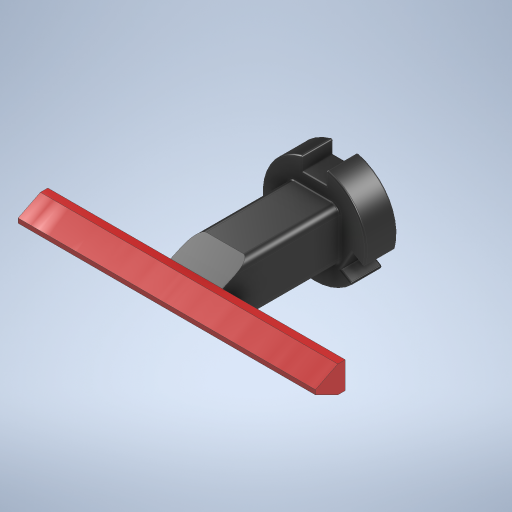
# Autodesk Inventor part: Squeegee
Saved by Autodesk Inventor 2023 (Build 270158000, 158)
## iProperties
Created: 2022-09-20
Part Number: Squeegee
Material: Generic
Document SubType Name: Modeling
Designer: benni
Density: 1 g/cm^3
Appearance: Default
Author: benni
Autodesk Inventor part; units mm, degrees
ref_plane "YZ Plane" through (0, 0, 0) normal (1, 0, 0) x (0, 1, 0)
ref_plane "XZ Plane" through (0, 0, 0) normal (0, 1, 0) x (-1, 0, 0)
ref_plane "XY Plane" through (0, 0, 0) normal (0, 0, 1) x (1, 0, 0)
sketch "Sketch1" plane through (0, 0, 0) normal (0, 0, 1) x (1, 0, 0)
  circle A0 centre (0, 0) radius 25 construction
  line L0 (0, 0) -> (0, 25) construction
  line L1 (0, 0) -> (21.6506, -12.5) construction
  line L2 (0, 0) -> (-21.6506, -12.5) construction
  line L3 (0, 25) -> (8, 25)
  line L4 (0, 25) -> (-8, 25)
  line L5 (0, 25) -> (8, 25) construction
  line L6 (21.6506, -12.5) -> (25.6506, -5.5718)
  line L7 (21.6506, -12.5) -> (29.6506, -12.5) construction
  line L8 (21.6506, -12.5) -> (17.6506, -19.4282)
  line L9 (21.6506, -12.5) -> (29.6506, -12.5) construction
  line L10 (-21.6506, -12.5) -> (-25.6506, -5.5718)
  line L11 (-21.6506, -12.5) -> (-13.6506, -12.5) construction
  line L12 (-21.6506, -12.5) -> (-17.6506, -19.4282)
  line L13 (-21.6506, -12.5) -> (-13.6506, -12.5) construction
  line L14 (8, 25) -> (8, 34.0735)
  line L15 (-8, 25) -> (-8, 34.0735)
  line L16 (25.6506, -5.5718) -> (33.5085, -10.1085)
  line L17 (17.6506, -19.4282) -> (25.5085, -23.9649)
  line L18 (-17.6506, -19.4282) -> (-25.5085, -23.9649)
  line L19 (-25.6506, -5.5718) -> (-33.5085, -10.1085)
  arc A1 (33.5085, -10.1085) -> (8, 34.0735) centre (0, 0) ccw
  arc A2 (-8, 34.0735) -> (-33.5085, -10.1085) centre (0, 0) ccw
  arc A3 (-25.5085, -23.9649) -> (25.5085, -23.9649) centre (0, 0) ccw
  dimension "d0" = 50
  dimension "d1" = 120
  dimension "d2" = 120
  dimension "d3" = 8
  dimension "d4" = 8
  dimension "d5" = 180
  dimension "d6" = 8
  dimension "d7" = 60
  dimension "d8" = 8
  dimension "d9" = 120
  dimension "d10" = 8
  dimension "d11" = 120
  dimension "d12" = 8
  dimension "d13" = 60
  dimension "d15" = 35
  dimension "d16" = 35
  dimension "d17" = 35
  constraints: 40 end point, 9 point on circle, 6 horizontal, 5 equal length, 4 centre point, 4 tangent, 3 parallel, 2 coincident, 2 perpendicular, 2 vertical, 1 collinear
  measures "d0" diameter of A0
  measures "d1" angle of L1 L0
  measures "d2" angle of L2 L1
  measures "d3" distance of L0.end L3.end
  measures "d4" distance of L0.end L4.end
  measures "d5" angle of L4 L5
  measures "d6" distance of L1.end L6.end
  measures "d7" angle of L7 L6
  measures "d8" distance of L1.end L8.end
  measures "d9" angle of L8 L9
  measures "d10" distance of L2.end L10.end
  measures "d11" angle of L11 L10
  measures "d12" distance of L2.end L12.end
  measures "d13" angle of L12 L13
  measures "d15" radius of A1
  measures "d16" radius of A2
  measures "d17" radius of A3
extrude "Extrusion1" add sketch "Sketch1" along normal blind 21
sketch "Sketch2" plane through (0, 0, 21) normal (0, 0, 1) x (1, 0, 0)
  line L0 (-17.5, -17.5) -> (17.5, -17.5)
  line L1 (17.5, -17.5) -> (17.5, 17.5)
  line L2 (17.5, 17.5) -> (-17.5, 17.5)
  line L3 (-17.5, 17.5) -> (-17.5, -17.5)
  line L4 (-17.5, -17.5) -> (17.5, 17.5) construction
  line L5 (17.5, -17.5) -> (-17.5, 17.5) construction
  point P0 (0, 0)
  dimension "d20" = 35
  dimension "d21" = 35
  constraints: 12 end point, 2 midpoint, 2 parallel, 1 horizontal, 1 perpendicular
  measures "d20" distance of L2.end L1.end
  measures "d21" distance of L1.end L0.end
extrude "Extrusion2" add sketch "Sketch2" along normal blind 79
fillet "Fillet1" radius 5 4 edges at (17.5, 17.5, 60.5) (17.5, -17.5, 60.5) (-17.5, 17.5, 60.5) (-17.5, -17.5, 60.5)
fillet "Fillet2" radius 1 37 edges at (30.3109, 17.5, 0) (-30.3109, 17.5, 0) (0, -35, 0) (21.6506, -12.5, 0) (29.5796, -7.8402, 0) (21.5796, -21.6966, 0) (8, 29.5367, 0) (0, 25, 0) (-8, 29.5367, 0) (-29.5796, -7.8402, 0) (-21.6506, -12.5, 0) (-21.5796, -21.6966, 0) (16.0355, 16.0355, 21) (17.5, 0, 21) (16.0355, -16.0355, 21) (0, -17.5, 21) (-16.0355, -16.0355, 21) (-17.5, 0, 21) (-16.0355, 16.0355, 21) (0, 17.5, 21) (0, 25, 21) (8, 29.5367, 21) (30.3109, 17.5, 21) (8, 34.0735, 10.5) (-8, 34.0735, 10.5) (-30.3109, 17.5, 21) (21.6506, -12.5, 21) (29.5796, -7.8402, 21) (33.5085, -10.1085, 10.5) (21.5796, -21.6966, 21) (25.5085, -23.9649, 10.5) (0, -35, 21) (-21.5796, -21.6966, 21) (-21.6506, -12.5, 21) (-29.5796, -7.8402, 21) (-33.5085, -10.1085, 10.5) (-25.5085, -23.9649, 10.5)
sketch "Sketch4" plane through (0, 0, 100) normal (0, 0, 1) x (1, 0, 0)
  line L0 (-100, 9) -> (100, 9)
  line L1 (100, 9) -> (100, -9)
  line L2 (100, -9) -> (-100, -9)
  line L3 (-100, -9) -> (-100, 9)
  line L4 (-100, 9) -> (100, -9) construction
  line L5 (100, 9) -> (-100, -9) construction
  point P0 (0, 0)
  dimension "d29" = 200
  dimension "d30" = 18
  constraints: 12 end point, 2 midpoint, 2 parallel, 1 horizontal, 1 perpendicular
  measures "d29" distance of L1.end L2.end
  measures "d30" distance of L0.end L1.end
extrude "Extrusion4" add sketch "Sketch4" along normal blind 20
chamfer "Chamfer1" distance 15 distance2 7.5 1 edges at (0, 9, 120) measured on face at (-5.8333, 9, 113.3333)
chamfer "Chamfer2" distance 15 distance2 7.5 1 edges at (0, -9, 120) measured on face at (5.8333, -9, 113.3333)
sketch "Sketch5" plane through (-17.5, -12.5, 22) normal (-1, 0, 0) x (0, 0, 1)
  line L0 (78, 25) -> (78, 21.5) projected
  line L1 (78, 21.5) -> (59, 30)
  line L2 (78, 30) -> (0, 30) projected
  line L3 (78, 21.5) -> (78, 3.5) projected
  line L4 (78, 3.5) -> (59, -5)
  line L5 (0, -5) -> (78, -5) projected
  line L6 (-1, 45.5377) -> (-1, 3.9006) projected
  line L7 (-1, -11.6878) -> (-1, -21.5) projected
  line L8 (59, 30) -> (79.7538, 33.0683)
  line L9 (79.7538, 33.0683) -> (78, 21.5)
  line L10 (78, 0) -> (78, 3.5) projected
  line L11 (78, 3.5) -> (84.2924, -8.3159)
  line L12 (84.2924, -8.3159) -> (59, -5)
  point P0 (-22, 12.5)
  dimension "d39" = 60
  dimension "d40" = 60
  constraints: 12 end point, 2 point on line
  measures "d39" distance from line of L1.end L6
  measures "d40" distance from line of L7 L4.end
extrude "Extrusion5" cut sketch "Sketch5" against normal through all
equation "\"d3\" = d4"
equation "\"d6\" = d4"
equation "\"d8\" = d4"
equation "\"d10\" = d4"
equation "\"d12\" = d4"
equation "\"d16\" = d15"
equation "\"d17\" = d15"
equation "\"d40\" = d39"
body "Solid1"
